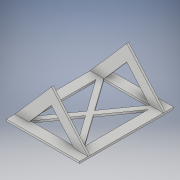
# Autodesk Inventor part: Square Support
Saved by Autodesk Inventor 2019 (Build 230136000, 136)
## iProperties
Created: 2019-04-16
Part Number: Square Support
Material: Generic
Document SubType Name: Modeling
Designer: kyle.fuchs
Density: 1 g/cm^3
Appearance: Default
Author: kyle.fuchs
Autodesk Inventor part; units mm, degrees
ref_plane "YZ Plane" through (0, 0, 0) normal (1, 0, 0) x (0, 1, 0)
ref_plane "XZ Plane" through (0, 0, 0) normal (0, 1, 0) x (-1, 0, 0)
sketch "Sketch1" plane through (0, 0, 0) normal (0, 1, 0) x (-1, 0, 0)
  line L0 (59.0386, -55.7993) -> (59.0386, -367.6994)
  line L1 (74.6457, -389.5494) -> (297.4316, -389.5494)
  line L2 (313.0386, -367.6994) -> (313.0386, -55.7993)
  line L3 (297.4316, -33.9494) -> (74.6457, -33.9494)
  line L4 (363.8386, 16.8506) -> (363.8386, -440.3494)
  line L5 (363.8386, -440.3494) -> (8.2386, -440.3494)
  line L6 (8.2386, -440.3494) -> (8.2386, 16.8506)
  line L7 (8.2386, 16.8506) -> (363.8386, 16.8506)
  line L8 (313.0386, -367.6994) -> (201.6457, -211.7494)
  line L9 (186.0386, -189.8994) -> (74.6457, -33.9494)
  line L10 (297.4316, -33.9494) -> (186.0386, -189.8994)
  line L11 (170.4316, -211.7494) -> (59.0386, -367.6994)
  line L12 (297.4316, -389.5494) -> (186.0386, -233.5993)
  line L13 (170.4316, -211.7494) -> (59.0386, -55.7993)
  line L14 (313.0386, -55.7993) -> (201.6457, -211.7494)
  line L15 (186.0386, -233.5993) -> (74.6457, -389.5494)
  point P0 (0, 0)
  dimension "d3" = 50.8
  constraints: 32 end point, 4 perpendicular, 1 vertical
  measures "d3" distance between parallel lines of L2 L4
extrude "Extrusion1" add sketch "Sketch1" along normal blind 9.525
sketch "Sketch5" plane through (-74.6457, 0, -33.9494) normal (0, 0, -1) x (-1, 0, 0)
  line L0 (0, 9.525) -> (222.7858, 9.525) projected
  line L1 (111.3929, 212.725) -> (-66.4071, 9.525)
  line L2 (111.3929, 212.725) -> (289.1929, 9.525)
  line L3 (1.0944, 9.525) -> (111.3929, 135.5805)
  line L4 (111.3929, 135.5805) -> (221.6915, 9.525)
  line L5 (-66.4071, 9.525) -> (1.0944, 9.525)
  line L6 (221.6915, 9.525) -> (289.1929, 9.525)
  point P0 (-74.6457, 0)
  dimension "d12" = 50.8
  constraints: 12 end point, 4 point on line, 1 collinear
  measures "d12" distance between parallel lines of L1 L3
extrude "Extrusion2" add sketch "Sketch5" against normal blind 9.525 contours L5 L1 L2 L6 L0 L4 L3
ref_plane "Work Plane1" through (0, 0, -212.09) normal (0, 0, 1) x (1, 0, 0)
mirror "Mirror1" about plane through (0, 0, -212.09) normal (0, 0, 1) of "Extrusion2"
body "Solid1"
